Autodesk Fusion 360 part; units mm, degrees
(part 2 of 3)
sketch "Sketch1" plane through (0, 0, 0) normal (0, 0, 1) x (1, 0, 0)
  line L0 (40, 31) -> (-40, 31)
  line L1 (-40, -31) -> (40, -31)
  line L2 (50, 31) -> (-50, -31) construction
  line L3 (-50, 31) -> (50, -31) construction
  line L4 (151, 31) -> (151, 141)
  line L5 (141, 151) -> (60, 151)
  line L6 (50, 141) -> (50, 41)
  line L7 (151, -31) -> (151, -141)
  line L8 (141, -151) -> (60, -151)
  line L9 (50, -141) -> (50, -41)
  line L10 (151, -31) -> (151, 31)
  line L11 (0, 0) -> (0, 31) construction
  line L12 (-141, 151) -> (-60, 151)
  line L13 (-50, 141) -> (-50, 41)
  line L14 (-151, 31) -> (-151, 141)
  line L15 (-151, -31) -> (-151, 31)
  line L16 (-141, -151) -> (-60, -151)
  line L17 (-50, -141) -> (-50, -41)
  line L18 (-151, -31) -> (-151, -141)
  circle A0 centre (0, 0) radius 5
  arc A1 (-141, 151) -> (-151, 141) centre (-141, 141) ccw
  arc A2 (-50, 141) -> (-60, 151) centre (-60, 141) ccw
  arc A3 (60, 151) -> (50, 141) centre (60, 141) ccw
  arc A4 (151, 141) -> (141, 151) centre (141, 141) ccw
  arc A5 (-151, -141) -> (-141, -151) centre (-141, -141) ccw
  arc A6 (-60, -151) -> (-50, -141) centre (-60, -141) ccw
  arc A7 (50, -141) -> (60, -151) centre (60, -141) ccw
  arc A8 (141, -151) -> (151, -141) centre (141, -141) ccw
  arc A9 (-40, -31) -> (-50, -41) centre (-40, -41) ccw
  arc A10 (50, -41) -> (40, -31) centre (40, -41) ccw
  arc A11 (40, 31) -> (50, 41) centre (40, 41) ccw
  arc A12 (-50, 41) -> (-40, 31) centre (-40, 41) ccw
  line L19 (100.5, -151) -> (100.5, -121) construction
  line L20 (119.25, -121) -> (81.75, -121) construction
  circle A13 centre (119.25, -121) radius 1.5
  circle A14 centre (81.75, -121) radius 1.5
  line L21 (151, 0) -> (100, 0) construction
  circle A15 centre (81.75, 121) radius 1.5
  circle A16 centre (119.25, 121) radius 1.5
  line L22 (0, -150) -> (0, -125) construction
  circle A17 centre (-81.75, -121) radius 1.5
  circle A18 centre (-119.25, -121) radius 1.5
  circle A19 centre (-81.75, 121) radius 1.5
  circle A20 centre (-119.25, 121) radius 1.5
  point P0 (50, 151)
  point P1 (50, -151)
  dimension "d1" = 100
  dimension "d2" = 62
  dimension "d3" = 101
  dimension "d4" = 120
  dimension "d5" = 101
  dimension "d6" = 120
  dimension "d9" = 10
  dimension "d10" = 10
  dimension "d11" = 30
  dimension "d12" = 18.75
  dimension "d13" = 37.5
  dimension "d14" = 3
  dimension "d15" = 3
  dimension "d21" = 51
  dimension "d22" = 25
  dimension "d23" = 125
  constraint horizontal L0
  constraint parallel L0 L1
  constraint coincident L2 L11.start
  constraint coincident L3 L11.start
  constraint coincident L11.start A0.centre
  constraint vertical L4
  constraint horizontal L5
  constraint vertical L6
  constraint vertical L7
  constraint horizontal L8
  constraint vertical L9
  constraint symmetric L4.start L11 L14.start
  constraint symmetric L7.start L11 L15.start
  constraint tangent L12 A1
  constraint tangent L14 A1
  constraint tangent L12 A2
  constraint tangent L13 A2
  constraint equal A1 A2
  constraint coincident P0 L5
  constraint coincident P0 L6
  constraint tangent L5 A3
  constraint tangent L6 A3
  constraint equal A1 A3
  constraint tangent L4 A4
  constraint tangent L5 A4
  constraint equal A1 A4
  constraint tangent L16 A5
  constraint tangent L18 A5
  constraint equal A1 A5
  constraint tangent L16 A6
  constraint tangent L17 A6
  constraint equal A1 A6
  constraint coincident P1 L8
  constraint coincident P1 L9
  constraint tangent L8 A7
  constraint tangent L9 A7
  constraint equal A1 A7
  constraint tangent L7 A8
  constraint tangent L8 A8
  constraint equal A1 A8
  constraint coincident L2.end L1
  constraint tangent L1 A9
  constraint tangent L17 A9
  constraint equal A1 A9
  constraint coincident L3.end L1
  constraint coincident L3.end L9
  constraint tangent L1 A10
  constraint tangent L9 A10
  constraint equal A1 A10
  constraint coincident L0 L11.end
  constraint coincident L2.start L6
  constraint coincident L2.start L0
  constraint tangent L6 A11
  constraint tangent L0 A11
  constraint equal A1 A11
  constraint coincident L3.start L0
  constraint tangent L13 A12
  constraint tangent L0 A12
  constraint equal A1 A12
  constraint midpoint L8 L19.start
  constraint perpendicular L8 L19
  constraint coincident L20.start A13.centre
  constraint coincident L20.end A14.centre
  constraint midpoint L10 L21.start
  constraint perpendicular L10 L21
  constraint symmetric A13 L21 A16
  constraint symmetric A14 L21 A15
  constraint vertical L22
  constraint symmetric A13 L22 A18
  constraint symmetric A14 L22 A17
  constraint symmetric A15 L22 A19
  constraint symmetric A16 L22 A20
  constraint parallel L14 L18
  constraint parallel L4 L17
  constraint parallel L1 L12
  constraint parallel L7 L14
  constraint parallel L4 L10
  constraint parallel L4 L13
  constraint parallel L4 L15
  constraint parallel L5 L16
  constraint collinear L5 L12
  constraint collinear L6 L9
  constraint collinear L8 L16
  constraint collinear L11 L22
  constraint collinear L13 L17
  constraint horizontal L20
  constraint vertical L2.end L17.start
  constraint vertical L3.start L17.start
  constraint horizontal L2.start L4.start
  constraint horizontal L19.end A18.centre
  constraint horizontal L11.start L21.end
  measures "d1" distance of L2.end L3.end
  measures "d2" distance of L3.start L2.end
  measures "d3" distance of L2.start L4.start
  measures "d4" distance of L2.start P0
  measures "d5" distance of L3.end L7.start
  measures "d6" distance of L3.end P1
  measures "d9" diameter of A0
  measures "d10" radius of A1
  measures "d11" distance of L19.start L19.end
  measures "d12" distance of L19.end L20.start
  measures "d13" distance of L20.start L20.end
  measures "d14" diameter of A13
  measures "d15" diameter of A14
  measures "d21" distance of L4 L21.end
  measures "d22" vertical distance of L22.start L22.end
  measures "d23" vertical distance of L11.start L22.end
extrude "Extrude1" add sketch "Sketch1" along normal blind 30.6
chamfer "Chamfer1" distance 5.2024 angle 41 1 edges at (-4.6616, 1.8081, 0) measured on face at (4.9938, -0.2492, 20.4)
extrude "Extrude2" cut 1 faces at (-96.5316, 12.7276, 30.6) along direction (0, 0, -1) blind 25.4
equation "d7 = 5.2 mm + 1 in"
equation "d12 = ( 37.5 / 2 ) * 1 mm"

design "FA6 - 12 Gauge 4” Staple Stake"
Autodesk Fusion 360 part; units mm, degrees
sketch "Sketch1" plane through (0, 0, 0) normal (0, 1, 0) x (1, 0, 0)
  line L0 (0, 0) -> (0, -101.6) construction
  line L1 (0, -101.6) -> (16.1278, -101.6)
  line L2 (18.6263, -99.1872) -> (22.09, 0)
  line L3 (18.542, -101.6) -> (48.3661, -101.6) construction
  line L4 (0, 0) -> (22.09, 0) construction
  arc A0 (16.1278, -101.6) -> (18.6263, -99.1872) centre (16.1278, -99.1) ccw
  line L5 (0, -101.6) -> (-16.1278, -101.6)
  arc A1 (-18.6263, -99.1872) -> (-16.1278, -101.6) centre (-16.1278, -99.1) ccw
  line L6 (-18.6263, -99.1872) -> (-22.09, 0)
  line L7 (0, -101.6) -> (-18.75, -101.6) construction
  line L8 (-18.75, -101.6) -> (-18.75, -100.3) construction
  dimension "d1" = 101.6
  dimension "d2" = 18.542
  dimension "d3" = 88
  dimension "d4" = 2.5
  dimension "d13" = 18.75
  dimension "d14" = 1.3
  constraint coincident L0.start L4.start
  constraint vertical L0
  constraint perpendicular L0 L1
  constraint horizontal L3
  constraint perpendicular L0 L4
  constraint coincident L3.start L1
  constraint coincident L3.start L2
  constraint tangent L1 A0
  constraint tangent L2 A0
  constraint symmetric L1.start L0 L5.start
  constraint symmetric L0 L2.end L6.end
  constraint symmetric L0 L1.end L5.end
  constraint symmetric L0 L2.start A1.start
  constraint symmetric L0 A0 A1
  constraint perpendicular L0 L7
  constraint perpendicular L7 L8
  measures "d1" distance of L0.start L0.end
  measures "d2" distance of L0.end L3.start
  measures "d3" angle of L2 L3
  measures "d4" radius of A0
  measures "d13" distance of L0.end L7.end
  measures "d14" distance of L7.end L8.end
sketch "Sketch3" plane through (0, 0, 0) normal (1, 0, 0) x (0, 1, 0)
  line L0 (0, 0) -> (0, 101.6) construction
  circle A0 centre (0, 101.6) radius 1.3
  dimension "d5" = 101.6
  dimension "d6" = 2.6
  constraint coincident L0.start origin
  constraint vertical L0
  constraint coincident L0.end A0.centre
  measures "d5" distance of L0.start L0.end
  measures "d6" diameter of A0
sweep "Sweep1" add profiles "Sketch3" path "Sketch1" along L6 A1 L5 L1 A0 L2 section 1
ref_plane "WorkPlane1" through (0, 0, 100.3) normal (0, 0, 1) x (1, 0, 0)
sketch "Sketch4" plane through (0, 0, 100.3) normal (0, 0, 1) x (1, 0, 0)
  line L0 (0, 0) -> (-18.75, 0) construction
  circle A0 centre (-18.75, 0) radius 5 construction
  dimension "d16" = 18.75
  dimension "d17" = 10
  constraint coincident L0.start origin
  constraint horizontal L0
  constraint coincident L0.end A0.centre
  measures "d16" distance of L0.start L0.end
  measures "d17" diameter of A0
chamfer "Chamfer1" distance 1.3 distance2 4 2 edges at (-22.5598, -1.212, 0.0164) (21.6201, -1.212, -0.0164) measured on face at (-22.2737, 0.4465, 0.0064) measured on face at (22.1502, -0.4097, 0.0021)
equation "d2 = ( 37.084 / 2 ) * 1 mm"
equation "d13 = ( 37.5 / 2 ) * 1 mm"

design "LB2 - Buffer Disk"
Autodesk Fusion 360 part; units mm, degrees
sketch "Sketch1" plane through (0, 0, 0) normal (0, 0, 1) x (1, 0, 0)
  circle A0 centre (0, 0) radius 31
  circle A1 centre (0, 0) radius 5
  dimension "d1" = 62
  dimension "d2" = 10
  constraint coincident A0.centre A1.centre
  constraint concentric A0 A1
  measures "d1" diameter of A0
  measures "d2" diameter of A1
extrude "Extrude1" add sketch "Sketch1" along normal blind 5.2

design "PE4 - PCB Case Lid"
Autodesk Fusion 360 part; units mm, degrees
sketch "Sketch1" plane through (0, 0, 0) normal (0, 0, 1) x (1, 0, 0)
  line L0 (6.2013, 11.75) -> (-6.2012, 11.75)
  line L1 (10.25, 10.25) -> (-10.25, -10.25) construction
  arc A0 (-6.2012, 11.75) -> (-11.75, 6.2013) centre (-6.2013, 6.2013) ccw
  line L2 (-11.75, 6.2013) -> (-11.75, -6.2013)
  arc A1 (-11.75, -6.2012) -> (-6.2012, -11.75) centre (-6.2013, -6.2013) ccw
  line L3 (-6.2012, -11.75) -> (6.2013, -11.75)
  arc A2 (11.75, 6.2012) -> (6.2013, 11.75) centre (6.2012, 6.2012) ccw
  arc A3 (6.2013, -11.75) -> (11.75, -6.2012) centre (6.2013, -6.2013) ccw
  line L4 (-10.25, 10.25) -> (10.25, -10.25) construction
  line L5 (11.75, -6.2012) -> (11.75, 6.2012)
  circle A4 centre (6.2012, 6.2012) radius 1.7
  circle A5 centre (-6.2013, -6.2013) radius 1.7
  line L6 (-6.2013, -6.2013) -> (-6.2013, -4) construction
  line L7 (-6.2013, -6.2013) -> (-4, -6.2013) construction
  line L8 (-4, -6.2013) -> (-4, -10.15)
  line L9 (-6.2013, -4) -> (-10.15, -4)
  line L10 (-4, -6.2013) -> (-4, -5)
  line L11 (-6.2013, -4) -> (-5, -4)
  arc A6 (-4, -5) -> (-5, -4) centre (-5, -5) ccw
  line L12 (6.2013, 4) -> (10.15, 4)
  line L13 (6.2013, 4) -> (5, 4)
  arc A7 (4, 5) -> (5, 4) centre (5, 5) ccw
  line L14 (4, 6.2013) -> (4, 5)
  line L15 (4, 6.2013) -> (4, 10.15)
  line L16 (10.15, -6.2012) -> (10.15, 6.2012)
  arc A8 (10.15, 6.2012) -> (6.2013, 10.15) centre (6.2012, 6.2012) ccw
  line L17 (6.2012, 10.15) -> (-6.2012, 10.15)
  arc A9 (-6.2012, 10.15) -> (-10.15, 6.2013) centre (-6.2013, 6.2013) ccw
  line L18 (-10.15, 6.2013) -> (-10.15, -6.2012)
  arc A10 (-10.15, -6.2012) -> (-6.2012, -10.15) centre (-6.2013, -6.2013) ccw
  line L19 (-6.2012, -10.15) -> (6.2013, -10.15)
  arc A11 (6.2013, -10.15) -> (10.15, -6.2013) centre (6.2013, -6.2013) ccw
  arc A12 (9.15, 6.2012) -> (6.2012, 9.15) centre (6.2012, 6.2012) ccw
  line L20 (6.2012, 9.15) -> (-6.2012, 9.15)
  arc A13 (-6.2012, 9.15) -> (-9.15, 6.2013) centre (-6.2013, 6.2013) ccw
  line L21 (-9.15, 6.2013) -> (-9.15, -6.2012)
  arc A14 (-9.15, -6.2012) -> (-6.2013, -9.15) centre (-6.2013, -6.2013) ccw
  line L22 (-6.2013, -9.15) -> (6.2013, -9.15)
  arc A15 (6.2013, -9.15) -> (9.15, -6.2013) centre (6.2013, -6.2013) ccw
  line L23 (9.15, -6.2013) -> (9.15, 6.2012)
  dimension "d2" = 20.5
  dimension "d3" = 20.5
  dimension "d8" = 3.4
  dimension "d9" = 3.4
  dimension "d13" = 1
  dimension "d26" = -1.6
  dimension "d27" = -2.6
  dimension "d89" = 5
  dimension "d90" = 9
  dimension "d91" = 9
  dimension "d92" = 6.75
  dimension "d93" = 1.2012
  dimension "d94" = 1
  dimension "d95" = 14.15
  dimension "d96" = 6.75
  dimension "d97" = 1.2012
  dimension "d98" = 14.15
  dimension "d99" = 2.2012
  dimension "d100" = 2.2012
  dimension "d101" = 2.2012
  dimension "d102" = 2.2012
  dimension "d103" = 135
  dimension "d104" = 5
  constraint coincident origin L1
  constraint coincident origin L4
  constraint vertical L6
  constraint perpendicular L6 L7
  constraint perpendicular L6 L9
  constraint perpendicular L7 L10
  constraint perpendicular L10 L11
  constraint tangent L10 A6
  constraint tangent L11 A6
  constraint vertical L15
  constraint horizontal L12
  constraint coincident L8.end L19
  constraint perpendicular L8 L19
  constraint coincident L9.end L18
  constraint perpendicular L9 L18
  constraint coincident L15.end L17
  constraint perpendicular L15 L17
  constraint coincident L12.end L16
  constraint perpendicular L12 L16
  constraint tangent A7 L14
  constraint tangent L13 A7
  constraint equal A6 A7
  constraint tangent A0 L2
  constraint tangent L0 A0
  constraint equal A0 A1
  constraint equal A0 A2
  constraint equal A0 A3
  constraint equal L10 L13
  constraint equal L10 L14
  constraint parallel L14 L15
  constraint parallel L12 L13
  constraint vertical L12.start L22.end
  constraint horizontal L14.start A12.start
  constraint midpoint origin L1
  constraint tangent L2 A1
  constraint equal L0 L2
  constraint equal L0 L18
  constraint equal L0 L21
  constraint equal L6 L7
  constraint equal L0 L23
  constraint equal L0 L16
  constraint equal L0 L5
  constraint tangent A1 L3
  constraint equal L0 L3
  constraint equal L0 L19
  constraint equal L0 L22
  constraint concentric A2 A4
  constraint concentric A1 A5
  constraint vertical L1.end L4.start
  constraint vertical L1.start L4.end
  constraint coincident A1.centre A5.centre
  measures "d2" distance of L1.start L4.start
  measures "d3" distance of L1.start L4.end
  measures "d8" diameter of A4
  measures "d9" diameter of A5
  measures "d13" radius of A6
  measures "d89" horizontal distance of origin A6.centre
  measures "d90" distance of A6.centre L13
  measures "d91" distance of A6.centre L14
  measures "d92" distance of L2 A6.centre
  measures "d93" distance of L6 A6.centre
  measures "d94" distance of L8 A6.centre
  measures "d95" distance of A6.centre L23
  measures "d96" distance of L3 A6.centre
  measures "d97" distance of L7 A6.centre
  measures "d98" distance of A6.centre L20
  measures "d99" distance of A0.centre L10
  measures "d100" distance of A3.centre L11
  measures "d101" distance of A2.centre L14
  measures "d102" distance of A2.centre L12
  measures "d103" angle of L1 L9
  measures "d104" vertical distance of origin A6.centre
sketch "Sketch2" plane through (0, 0, 0) normal (0, 0, 1) x (1, 0, 0)
  line L0 (-6.2013, -27.25) -> (6.2012, -27.25)
  arc A0 (6.2012, -27.25) -> (12.25, -21.2012) centre (6.2013, -21.2012) ccw
  line L1 (12.25, -21.2012) -> (12.25, 21.2013)
  arc A1 (12.25, 21.2013) -> (6.2013, 27.25) centre (6.2012, 21.2013) ccw
  line L2 (6.2013, 27.25) -> (-6.2012, 27.25)
  arc A2 (-6.2012, 27.25) -> (-12.25, 21.2013) centre (-6.2013, 21.2013) ccw
  line L3 (-12.25, 21.2013) -> (-12.25, -21.2012)
  arc A3 (-12.25, -21.2012) -> (-6.2013, -27.25) centre (-6.2013, -21.2012) ccw
  line L4 (-10.15, 21.2013) -> (-10.15, -21.2012)
  arc A4 (-10.15, -21.2012) -> (-6.2013, -25.15) centre (-6.2013, -21.2012) ccw
  line L5 (-6.2013, -25.15) -> (6.2013, -25.15)
  arc A5 (6.2013, -25.15) -> (10.15, -21.2012) centre (6.2013, -21.2012) ccw
  line L6 (10.15, -21.2012) -> (10.15, 17.8428)
  line L7 (2.8428, 25.15) -> (-6.2013, 25.15)
  arc A6 (-6.2013, 25.15) -> (-10.15, 21.2013) centre (-6.2013, 21.2013) ccw
  circle A7 centre (6.9428, 21.9428) radius 1.6
  circle A8 centre (-6.9428, -21.9428) radius 1.6
  line L8 (-6.2013, -25.15) -> (6.2012, -25.15)
  arc A9 (6.2012, -25.15) -> (10.15, -21.2012) centre (6.2013, -21.2012) ccw
  line L9 (10.15, -21.2012) -> (10.15, 21.2013)
  arc A10 (10.15, 21.2013) -> (6.2013, 25.15) centre (6.2012, 21.2013) ccw
  line L10 (6.2013, 25.15) -> (-6.2012, 25.15)
  arc A11 (-6.2012, 25.15) -> (-10.15, 21.2013) centre (-6.2013, 21.2013) ccw
  line L11 (-10.15, 21.2013) -> (-10.15, -21.2012)
  arc A12 (-10.15, -21.2012) -> (-6.2013, -25.15) centre (-6.2013, -21.2012) ccw
  line L12 (2.8428, 23.65) -> (-6.2013, 23.65)
  arc A13 (-6.2013, 23.65) -> (-8.65, 21.2013) centre (-6.2013, 21.2013) ccw
  line L13 (-8.65, 21.2013) -> (-8.65, -17.8428)
  line L14 (2.8428, 25.15) -> (2.8428, 23.65)
  line L15 (-8.65, -17.8428) -> (-10.15, -17.8428)
  line L16 (-2.8428, -23.65) -> (6.2013, -23.65)
  arc A14 (6.2013, -23.65) -> (8.65, -21.2012) centre (6.2013, -21.2012) ccw
  line L17 (8.65, -21.2012) -> (8.65, 17.8428)
  line L18 (-2.8428, -25.15) -> (-2.8428, -23.65)
  line L19 (10.15, 17.8428) -> (8.65, 17.8428)
  dimension "d62" = 3.2
  dimension "d63" = 3.2
  dimension "d71" = -2.1
  dimension "d105" = 8.65
  dimension "d106" = 17.8428
  dimension "d107" = 1.7072
  dimension "d108" = 15.5928
  dimension "d109" = 4.1
  dimension "d110" = 39.7857
  dimension "d111" = 6.0488
  dimension "d112" = 1.5
  dimension "d113" = 39.0441
  dimension "d114" = 2.4487
  dimension "d115" = 2.4488
  dimension "d116" = 5.8072
  dimension "d117" = 11.4928
  dimension "d118" = 14.8513
  dimension "d119" = 17.3
  dimension "d120" = 18.8
  dimension "d121" = 9.4072
  dimension "d122" = 5.8072
  dimension "d123" = 35.6857
  dimension "d124" = 7.3072
  dimension "d125" = 22.4
  dimension "d126" = 1.5
  constraint coincident L5 L18.start
  constraint perpendicular L7 L14
  constraint perpendicular L11 L15
  constraint coincident L4 L15.end
  constraint perpendicular L16 L18
  constraint perpendicular L17 L19
  constraint tangent A14 L17
  constraint tangent A13 L13
  constraint tangent L7 A11
  constraint tangent L3 A3
  constraint tangent L0 A3
  constraint tangent A2 L3
  constraint tangent L2 A2
  constraint tangent A1 L2
  constraint tangent L1 A1
  constraint tangent L0 A0
  constraint tangent A0 L1
  constraint concentric A6 A11
  constraint concentric A11 A13
  constraint concentric A3 A4
  constraint concentric A0 A5
  constraint coincident L4.start A11
  constraint perpendicular L13 L15
  constraint perpendicular L4 L15
  constraint equal A0 A3
  constraint equal A0 A2
  constraint equal A0 A1
  constraint equal L6 L13
  constraint equal L14 L15
  constraint midpoint A6 A11
  constraint midpoint L4 L11
  constraint parallel L0 L12
  constraint equal L7 L16
  measures "d62" diameter of A7
  measures "d63" diameter of A8
  measures "d105" distance of origin L13
  measures "d106" distance of origin L15
  measures "d107" distance of A8.centre L13
  measures "d108" distance of A7.centre L13
  measures "d109" distance of A8.centre L15
  measures "d110" distance of A7.centre L15
  measures "d111" radius of A2
  measures "d112" distance of L4.start L13
  measures "d113" distance of L1.end L15
  measures "d114" distance of L0.start L13
  measures "d115" distance of L2.end L13
  measures "d116" distance of L13 L18
  measures "d117" distance of L13 L14
  measures "d118" distance of A1.end L13
  measures "d119" distance of L13 L17
  measures "d120" distance of L9 L13
  measures "d121" distance of L0 L15
  measures "d122" distance of L15 L16
  measures "d123" distance of L15 L19
  measures "d124" distance of L18.start L15
  measures "d125" distance of L3 L6
  measures "d126" distance of A5 A14
extrude "Extrude5" add sketch "Sketch2" along normal blind 5 contours L0 A0 L1 A1 L2 A2 L3 A3 | L4 L7 A6 L10 A11 L11 L12 A13 L13 L14 L15 | L4 A4 L5 L8 L9 A10 L10 L11 A12 L12 A13 L13 L14 L15 L16 A14 L17 L18 L19 | L5 A5 L6 L8 A9 L9 L16 A14 L17 L18 L19 | A7 | A8
extrude "Extrude6" add sketch "Sketch2" against normal blind 2 contours L4 L7 A6 L10 A11 L11 L12 A13 L13 L14 L15 | L5 A5 L6 L8 A9 L9 L16 A14 L17 L18 L19
sketch "Sketch3" plane through (0, 0, 0) normal (0, 1, 0) x (1, 0, 0)
  line L0 (1.7, 3) -> (1.7, 0) construction
  line L1 (-0.45, 0) -> (-0.45, 2.15)
  line L2 (3.85, -0.0044) -> (3.85, 2.1456)
  line L3 (-0.45, 2.15) -> (3.85, 2.1456)
  arc A0 (1.7991, 2.1477) -> (1.6052, 2.1479) centre (1.7, 0) ccw
  arc A1 (-0.45, 0) -> (3.85, 0.0044) centre (1.7, 0) ccw
  line L4 (5.2, -5) -> (-1.8, -5)
  line L5 (-1.8, -5) -> (-1.8, 0)
  line L6 (5.2, 0) -> (5.2, -5)
  line L7 (5.2, -5) -> (0.1955, 2.1493) construction
  line L8 (-1.8, -5) -> (3.2024, 2.1463) construction
  line L9 (5.2, 0) -> (3.85, 0)
  line L10 (-0.45, 0) -> (-1.8, 0)
  point P0 (1.7, 0)
  dimension "d45" = 2.15
  dimension "d46" = 2.15
  dimension "d127" = 2.15
  dimension "d128" = 3.5
  dimension "d129" = 3.5
  dimension "d130" = 2.15
  dimension "d131" = 1.5045
  dimension "d132" = 1.5024
  dimension "d133" = 0.45
  dimension "d134" = 8
  constraint vertical L0
  constraint coincident L1.start A0
  constraint vertical L1
  constraint coincident L2.start A0
  constraint vertical L2
  constraint coincident L2 A1.end
  constraint coincident L3 A0.start
  constraint coincident L3 A0.end
  constraint concentric A0 A1
  constraint horizontal L4
  constraint perpendicular L4 L5
  constraint parallel L5 L6
  constraint coincident L7 P0
  constraint coincident L8 P0
  constraint coincident P0 L0.end
  constraint horizontal L9
  constraint coincident L3 L8.end
  constraint coincident L3 L7.end
  constraint coincident L2 L9.end
  constraint collinear L9 L10
  constraint horizontal origin L1.start
  constraint tangent L1 A1
  measures "d45" distance of L1.start L1.end
  measures "d46" distance of L2.start L2.end
  measures "d127" radius of A1
  measures "d128" distance of L0 L5
  measures "d129" distance of L0 L6
  measures "d130" distance of L0 L2
  measures "d131" distance of L0 L7.end
  measures "d132" distance of L0 L8.end
  measures "d133" distance of origin L1
  measures "d134" distance of L0.start L4
extrude "Extrude7" cut sketch "Sketch2" along normal blind 3 contours L4 A4 L5 L8 L9 A10 L10 L11 A12 L12 A13 L13 L14 L15 L16 A14 L17 L18 L19 | A7 | A8
extrude "Extrude8" cut sketch "Sketch3" against normal blind 31 contours L1 L2 L3 A0 A1
extrude "Extrude9" add sketch "Sketch3" against normal blind 8 from surface at -27.25 contours L2 A1 L4 L5 L6 L9 L10
sketch "Sketch4" plane through (0, 0, 0) normal (0, 1, 0) x (1, 0, 0)
  line L0 (6.2012, 4) -> (6.2, 4)
  line L1 (-6.2013, 0) -> (0.8, 0)
  line L2 (-4.85, 0) -> (-4.85, 2.15)
  line L3 (-4.85, 2.15) -> (-0.55, 2.1456)
  line L4 (-0.55, -0.0044) -> (-0.55, 2.1456)
  line L5 (-4.85, 0) -> (-2.7, 0) construction
  arc A0 (-4.85, 0) -> (-0.55, 0.0044) centre (-2.7, 0) ccw
  arc A1 (-2.6009, 2.1477) -> (-2.7948, 2.1479) centre (-2.7, 0) ccw
  line L6 (-6.2, -5) -> (0.8, -5)
  line L7 (0.8, -5) -> (0.8, 0)
  line L8 (-6.2, 0) -> (-6.2, -5)
  line L9 (-6.2, -5) -> (-1.1976, 2.1463) construction
  line L10 (0.8, -5) -> (-4.2045, 2.1493) construction
  line L11 (-4.85, 0) -> (-6.2013, 0)
  line L12 (-0.55, -0.0044) -> (0.8, 0)
  point P0 (-2.7, 0)
  dimension "d53" = 2.15
  dimension "d54" = 2.15
  dimension "d55" = 2.15
  dimension "d135" = 0.55
  dimension "d136" = 6.75
  dimension "d137" = 2.15
  dimension "d138" = 0.0044
  dimension "d139" = 1.35
  dimension "d140" = 4.9956
  dimension "d141" = 5.65
  dimension "d142" = 6.7513
  dimension "d143" = 4
  dimension "d144" = 5.6512
  constraint horizontal L1
  constraint horizontal L0
  constraint vertical L2
  constraint vertical L4
  constraint perpendicular L2 L5
  constraint coincident L3 A1.end
  constraint coincident L4 A0.end
  constraint coincident L3 A1.start
  constraint concentric A0 A1
  constraint horizontal L6
  constraint perpendicular L6 L7
  constraint parallel L7 L8
  constraint coincident L9 P0
  constraint coincident L10 P0
  constraint coincident P0 L5.end
  constraint perpendicular L8 L11
  constraint coincident L3 L9.end
  constraint coincident L3 L10.end
  constraint coincident L1 L8.start
  constraint tangent L2 A0
  constraint coincident L4.start A0
  constraint equal A0 A1
  constraint coincident origin L1
  measures "d53" distance of L2.start L2.end
  measures "d54" distance of L3.end L4.start
  measures "d55" distance of L2.start P0
  measures "d135" distance of origin L4
  measures "d136" distance of L0.end L4
  measures "d137" radius of A0
  measures "d138" distance of L4.start L5
  measures "d139" distance of L4 L7
  measures "d140" distance of L4.start L6
  measures "d141" distance of L4 L8
  measures "d142" distance of L0.start L4
  measures "d143" distance of L0 L11
  measures "d144" distance of L1.start L4
extrude "Extrude10" add sketch "Sketch4" along normal blind 8 from surface at 27.25 contours L1 A0 L6 L7 L8 L11 L12
extrude "Extrude11" cut sketch "Sketch4" along normal blind 61 contours L1 L2 L3 L4 A0 A1 | L1 L4 A0
extrude "Extrude12" cut sketch "Sketch2" along normal blind 20 contours A7 | A8
extrude "Extrude13" add 1 faces at (-4.3101, 7.137, 5) along direction (0, 0, 1) blind 2
sketch "Sketch5" plane through (0, 0, 3) normal (0, 0, -1) x (1, 0, 0)
  circle A0 centre (6.9428, -21.9428) radius 1.6
  circle A1 centre (-6.9428, 21.9428) radius 1.6
  arc A2 (-6.2013, 25.15) -> (-10.15, 21.2012) centre (-6.2013, 21.2012) ccw
  line L0 (-10.15, 21.2012) -> (-10.15, 17.8428)
  line L1 (2.8428, -25.15) -> (6.2013, -25.15)
  arc A3 (6.2013, -25.15) -> (10.15, -21.2013) centre (6.2012, -21.2013) ccw
  line L2 (10.15, -21.2013) -> (10.15, -17.8428)
  line L3 (9.15, -17.8428) -> (-9.15, -17.8428)
  line L4 (-9.15, -17.8428) -> (-9.15, 17.8428)
  line L5 (-9.15, 17.8428) -> (9.15, 17.8428)
  line L6 (9.15, 17.8428) -> (9.15, -17.8428)
  line L7 (-10.15, 17.8428) -> (-8.65, 17.8428)
  line L8 (-8.65, 17.8428) -> (-8.65, -21.2013)
  arc A4 (-8.65, -21.2013) -> (-6.2013, -23.65) centre (-6.2013, -21.2013) ccw
  line L9 (-6.2013, -23.65) -> (2.8428, -23.65)
  line L10 (2.8428, -23.65) -> (2.8428, -25.15)
  line L11 (10.15, -17.8428) -> (8.65, -17.8428)
  line L12 (8.65, -17.8428) -> (8.65, 21.2012)
  arc A5 (8.65, 21.2012) -> (6.2013, 23.65) centre (6.2013, 21.2012) ccw
  line L13 (6.2013, 23.65) -> (-2.8428, 23.65)
  line L14 (-2.8428, 23.65) -> (-2.8428, 25.15)
  line L15 (-2.8428, 25.15) -> (-6.2013, 25.15)
  dimension "d145" = 1
  dimension "d146" = 18.3
  constraint horizontal L3
  constraint vertical L4
  constraint horizontal L5
  constraint vertical L6
  constraint coincident L3.start L11
  constraint coincident L4.end L7
  measures "d145" distance of L0.end L4
  measures "d146" distance of L4 L6
extrude "Extrude14" cut sketch "Sketch5" against normal blind 2 contours L3 L4 L5 L7 L8 | L3 L5 L8 L12 | L3 L5 L6 L11 L12
sketch "Sketch6" plane through (0, 0, 5) normal (0, 0, -1) x (1, 0, 0)
  line L0 (9.15, 17.8428) -> (-9.15, 17.8428)
  line L1 (-9.15, 17.8428) -> (-9.15, -17.8428)
  line L2 (-9.15, -17.8428) -> (9.15, -17.8428)
  line L3 (9.15, -17.8428) -> (9.15, 17.8428)
  line L4 (6.2012, -6.2012) -> (6.2012, -3.7012) construction
  line L5 (6.2012, -3.7012) -> (9.15, -3.7012)
  line L6 (9.15, -8.7012) -> (6.2012, -8.7012)
  arc A0 (6.2012, -3.7012) -> (6.2012, -8.7012) centre (6.2012, -6.2012) ccw
  line L7 (-6.2013, 3.7013) -> (-9.15, 3.7013)
  line L8 (-9.15, 8.7013) -> (-6.2013, 8.7013)
  arc A1 (-6.2013, 3.7013) -> (-6.2013, 8.7013) centre (-6.2013, 6.2013) ccw
  line L9 (-9.15, 3.7013) -> (-10.15, 3.7013)
  line L10 (-10.15, 3.7013) -> (-10.15, 8.7013)
  line L11 (-10.15, 8.7013) -> (-9.15, 8.7013)
  line L12 (9.15, -8.7012) -> (10.15, -8.7012)
  line L13 (10.15, -8.7012) -> (10.15, -3.7012)
  line L14 (10.15, -3.7012) -> (9.15, -3.7012)
  dimension "d75" = 5
  dimension "d76" = 5
  dimension "d79" = 1
  dimension "d80" = 5
  dimension "d81" = 1
  dimension "d82" = 5
  dimension "d147" = 15.3512
  dimension "d148" = 21.5441
  dimension "d149" = 14.1416
  constraint coincident L4.start A0.centre
  constraint parallel L5 L6
  constraint parallel L7 L8
  constraint horizontal L9
  constraint vertical L10
  constraint horizontal L11
  constraint horizontal L12
  constraint vertical L13
  constraint horizontal L14
  constraint tangent L7 A1
  constraint tangent L8 A1
  constraint tangent L6 A0
  constraint tangent L5 A0
  constraint coincident L1 L7.end
  constraint coincident L1 L8.start
  constraint coincident L3 L5.end
  constraint coincident L3 L6.start
  constraint equal L5 L7
  measures "d75" diameter of A1
  measures "d76" diameter of A0
  measures "d79" distance of L7.end L9.end
  measures "d80" distance of L7.end L8.start
  measures "d81" distance of L6.start L12.end
  measures "d82" distance of L6.start L5.end
  measures "d147" distance of L1 L4
  measures "d148" distance of L2 L7
  measures "d149" distance of L2 L5
extrude "Extrude15" add sketch "Sketch6" along normal blind 12.45 contours L3 L12 L13 L14 | L3 L5 L6 A0 | L1 L7 L8 A1 | L1 L9 L10 L11
extrude "Extrude16" add 1 faces at (-2.0372, -23.65, 0.4401) along direction (0, 1, 0) blind 2
extrude "Extrude17" add 1 faces at (1.7037, 23.65, 0.4415) along direction (0, -1, 0) blind 2
equation "d45 = ( 4.3 / 2 ) * 1 mm"
equation "d46 = ( 4.3 / 2 ) * 1 mm"
equation "d53 = ( 4.3 / 2 ) * 1 mm"
equation "d54 = ( 4.3 / 2 ) * 1 mm"
equation "d55 = ( 4.3 / 2 ) * 1 mm"
equation "d77 = 5.00 mm + 7.45 mm"

design "Top Component (FA1)"
Autodesk Fusion 360 part; units mm, degrees
sketch "Sketch1" plane through (0, 0, 0) normal (0, 0, 1) x (1, 0, 0)
  circle A0 centre (0, 0) radius 110
  circle A1 centre (0, 0) radius 106.5
  arc A2 (10.2564, 113.75) -> (12.5979, 109.2762) centre (20, 116) ccw
  arc A3 (9.7436, 118.25) -> (-10, 116) centre (0, 116) ccw
  arc A4 (-12.5979, 109.2762) -> (-10, 116) centre (-20, 116) ccw
  line L0 (0, 113.75) -> (10.2564, 113.75)
  line L1 (9.7436, 118.25) -> (0, 118.25)
  arc A5 (0, 118.25) -> (0, 113.75) centre (0, 116) ccw
  line L2 (12.5979, 109.2762) -> (12.5979, 107)
  line L3 (12.5979, 107) -> (-12.5979, 107)
  line L4 (-12.5979, 107) -> (-12.5979, 109.2762)
  dimension "d1" = 220
  dimension "d2" = 213
  dimension "d41" = 4.5
  dimension "d54" = 7.75
  dimension "d55" = 12.5979
  dimension "d56" = 107
  dimension "d57" = 11.25
  dimension "d58" = 40
  dimension "d59" = 10.2564
  constraint coincident A0.centre A1.centre
  constraint concentric A0 A1
  constraint parallel L0 L1
  constraint vertical L2
  constraint perpendicular L2 L3
  constraint perpendicular L3 L4
  constraint tangent L0 A5
  constraint tangent L1 A5
  constraint concentric A3 A5
  constraint coincident A0 A2.end
  constraint vertical A0.centre L0.start
  constraint equal A2 A3
  constraint equal A2 A4
  constraint coincident A3.end A4.end
  constraint parallel L0 L3
  constraint equal L2 L4
  measures "d1" diameter of A0
  measures "d2" diameter of A1
  measures "d41" diameter of A5
  measures "d54" distance of A3 A5
  measures "d55" distance of A0.centre L4
  measures "d56" distance of A0.centre L3
  measures "d57" distance of A3.start L3
  measures "d58" horizontal distance of A4.centre A2.centre
  measures "d59" distance of L0.start A2.start
ref_plane "WorkPlane1" through (0, 0, 220) normal (0, 0, 1) x (1, 0, 0)
sketch "Sketch2" plane through (0, 0, 220) normal (0, 0, 1) x (1, 0, 0)
  circle A0 centre (0, 0) radius 105
  circle A1 centre (0, 0) radius 101.5
  dimension "d4" = 210
  dimension "d5" = 203
  constraint coincident A0.centre A1.centre
  measures "d4" diameter of A0
  measures "d5" diameter of A1
sketch "Sketch3" plane through (0, 0, 0) normal (0, 1, 0) x (1, 0, 0)
  line L0 (0, 0) -> (-110, 0) construction
  line L1 (-110, 0) -> (-106.5, 0)
  line L2 (0, -200) -> (-105, -200) construction
  line L3 (-105, -200) -> (-101.5, -200)
  line L4 (-105, -200) -> (-110, 0)
  line L5 (-106.5, 0) -> (-101.5, -200)
  line L6 (0, 0) -> (0, -10) construction
  line L7 (0, -10) -> (0, -200) construction
  dimension "d6" = 110
  dimension "d7" = 3.5
  dimension "d8" = 105
  dimension "d9" = 3.5
  dimension "d42" = 190
  dimension "d60" = 200
  constraint coincident L0.start L6.start
  constraint horizontal L0
  constraint parallel L0 L1
  constraint horizontal L2
  constraint parallel L2 L3
  constraint perpendicular L0 L6
  constraint perpendicular L0 L7
  constraint coincident L2.start L7.end
  measures "d6" distance of L0.start L0.end
  measures "d7" distance of L0.end L1.end
  measures "d8" distance of L2.start L2.end
  measures "d9" distance of L2.end L3.end
  measures "d42" distance of L6.end L2.start
  measures "d60" distance of L0 L2
revolve "Revolve1" add sketch "Sketch3" angle 360 about axis through (0, 0, 1.75) along (0, 0, 1) makes body 1
extrude "Extrude1" add sketch "Sketch1" along normal blind 4 contours A0 L2 L3 L4 | A0 A2 A3 A4 L0 L1 A5 picked at (1.4025, 107.9732) bodies 1
pattern_circular "C-Pattern1" count 4 over 360 about axis through (0, 0, 1.75) along (0, 0, 1) of "Extrude1"
ref_plane "WorkPlane2" through (0, 0, 110) normal (0, 0, 1) x (1, 0, 0)
sketch "Sketch5" plane through (0, 0, 0) normal (0, 1, 0) x (-1, 0, 0)
  line L0 (-30, 114) -> (-103.6332, 140.8003)
  line L1 (-0.0018, 113.6676) -> (57.7728, 113.6676) construction
  line L2 (-103.6332, 140.8003) -> (-106.3694, 133.2828)
  line L3 (-106.3694, 133.2828) -> (-31.4106, 106)
  line L4 (-30, 114) -> (-30, 106)
  line L5 (-30, 106) -> (-31.4106, 106)
  line L6 (0, 0) -> (0, 110) construction
  point P0 (-30, 110)
  dimension "d47" = 30
  dimension "d49" = 160
  dimension "d50" = 8
  dimension "d51" = 8
  dimension "d52" = 110
  dimension "d61" = 0.3324
  dimension "d62" = 34.8003
  dimension "d63" = 57.7746
  constraint horizontal L1
  constraint perpendicular L0 L2
  constraint parallel L0 L3
  constraint perpendicular L4 L5
  constraint coincident L6.start origin
  constraint perpendicular L1 L6
  constraint midpoint L4 P0
  constraint vertical L4.end P0
  measures "d47" distance of L1.start L0.start
  measures "d49" angle of L0 L1
  measures "d50" distance of L0.end L2.end
  measures "d51" distance of L0.start L4.end
  measures "d52" distance of L6.start L6.end
  measures "d61" distance of L0.start L1
  measures "d62" vertical distance of L0.end L3.end
  measures "d63" horizontal distance of L1.start L1.end
sketch "Sketch4" plane through (0, 0, 110) normal (0, 0, 1) x (1, 0, 0)
  circle A0 centre (0, 0) radius 105.125
  circle A1 centre (0, 0) radius 30
  line L0 (2.5, 2.5) -> (-2.5, 2.5)
  line L1 (-2.5, 2.5) -> (-2.5, -2.5)
  line L2 (-2.5, -2.5) -> (2.5, -2.5)
  line L3 (2.5, -2.5) -> (2.5, 2.5)
  line L4 (2.5, 2.5) -> (-2.5, -2.5) construction
  line L5 (-2.5, 2.5) -> (2.5, -2.5) construction
  line L6 (-10, -27.5) -> (-10, -28.2843)
  line L7 (-5, -27.5) -> (-10, -27.5)
  line L8 (-5, -29.5804) -> (-5, -27.5)
  line L9 (-2.5, -27.5) -> (-2.5, -29.8957)
  line L10 (2.5, -27.5) -> (-2.5, -27.5)
  line L11 (2.5, -29.8957) -> (2.5, -27.5)
  line L12 (5, -27.5) -> (5, -29.5804)
  line L13 (10, -27.5) -> (5, -27.5)
  line L14 (10, -28.2843) -> (10, -27.5)
  line L15 (-20, -20) -> (-22.3607, -20)
  line L16 (-20, -22.3607) -> (-20, -20)
  line L17 (-17.5, -20) -> (-17.5, -24.367)
  line L18 (-16.5831, -25) -> (-12.5, -25)
  line L19 (-12.5, -20) -> (-17.5, -20)
  line L20 (-12.5, -25) -> (-12.5, -20)
  line L21 (-10, -20) -> (-10, -25)
  line L22 (-10, -25) -> (-5, -25)
  line L23 (-5, -20) -> (-10, -20)
  line L24 (-5, -25) -> (-5, -20)
  line L25 (-2.5, -20) -> (-2.5, -25)
  line L26 (-2.5, -25) -> (2.5, -25)
  line L27 (2.5, -20) -> (-2.5, -20)
  line L28 (2.5, -25) -> (2.5, -20)
  line L29 (5, -20) -> (5, -25)
  line L30 (5, -25) -> (10, -25)
  line L31 (10, -20) -> (5, -20)
  line L32 (10, -25) -> (10, -20)
  line L33 (12.5, -20) -> (12.5, -25)
  line L34 (12.5, -25) -> (16.5831, -25)
  line L35 (17.5, -20) -> (12.5, -20)
  line L36 (17.5, -24.367) -> (17.5, -20)
  line L37 (20, -20) -> (20, -22.3607)
  line L38 (22.3607, -20) -> (20, -20)
  line L39 (-25, -12.5) -> (-25, -16.5831)
  line L40 (-24.367, -17.5) -> (-20, -17.5)
  line L41 (-20, -12.5) -> (-25, -12.5)
  line L42 (-20, -17.5) -> (-20, -12.5)
  line L43 (-17.5, -12.5) -> (-17.5, -17.5)
  line L44 (-17.5, -17.5) -> (-12.5, -17.5)
  line L45 (-12.5, -12.5) -> (-17.5, -12.5)
  line L46 (-12.5, -17.5) -> (-12.5, -12.5)
  line L47 (-10, -12.5) -> (-10, -17.5)
  line L48 (-10, -17.5) -> (-5, -17.5)
  line L49 (-5, -12.5) -> (-10, -12.5)
  line L50 (-5, -17.5) -> (-5, -12.5)
  line L51 (-2.5, -12.5) -> (-2.5, -17.5)
  line L52 (-2.5, -17.5) -> (2.5, -17.5)
  line L53 (2.5, -12.5) -> (-2.5, -12.5)
  line L54 (2.5, -17.5) -> (2.5, -12.5)
  line L55 (5, -12.5) -> (5, -17.5)
  line L56 (5, -17.5) -> (10, -17.5)
  line L57 (10, -12.5) -> (5, -12.5)
  line L58 (10, -17.5) -> (10, -12.5)
  line L59 (12.5, -12.5) -> (12.5, -17.5)
  line L60 (12.5, -17.5) -> (17.5, -17.5)
  line L61 (17.5, -12.5) -> (12.5, -12.5)
  line L62 (17.5, -17.5) -> (17.5, -12.5)
  line L63 (20, -12.5) -> (20, -17.5)
  line L64 (20, -17.5) -> (24.367, -17.5)
  line L65 (25, -12.5) -> (20, -12.5)
  line L66 (25, -16.5831) -> (25, -12.5)
  line L67 (-28.2843, -10) -> (-27.5, -10)
  line L68 (-27.5, -5) -> (-29.5804, -5)
  line L69 (-27.5, -10) -> (-27.5, -5)
  line L70 (-25, -5) -> (-25, -10)
  line L71 (-25, -10) -> (-20, -10)
  line L72 (-20, -5) -> (-25, -5)
  line L73 (-20, -10) -> (-20, -5)
  line L74 (-17.5, -5) -> (-17.5, -10)
  line L75 (-17.5, -10) -> (-12.5, -10)
  line L76 (-12.5, -5) -> (-17.5, -5)
  line L77 (-12.5, -10) -> (-12.5, -5)
  line L78 (-10, -5) -> (-10, -10)
  line L79 (-10, -10) -> (-5, -10)
  line L80 (-5, -5) -> (-10, -5)
  line L81 (-5, -10) -> (-5, -5)
  line L82 (-2.5, -5) -> (-2.5, -10)
  line L83 (-2.5, -10) -> (2.5, -10)
  line L84 (2.5, -5) -> (-2.5, -5)
  line L85 (2.5, -10) -> (2.5, -5)
  line L86 (5, -5) -> (5, -10)
  line L87 (5, -10) -> (10, -10)
  line L88 (10, -5) -> (5, -5)
  line L89 (10, -10) -> (10, -5)
  line L90 (12.5, -5) -> (12.5, -10)
  line L91 (12.5, -10) -> (17.5, -10)
  line L92 (17.5, -5) -> (12.5, -5)
  line L93 (17.5, -10) -> (17.5, -5)
  line L94 (20, -5) -> (20, -10)
  line L95 (20, -10) -> (25, -10)
  line L96 (25, -5) -> (20, -5)
  line L97 (25, -10) -> (25, -5)
  line L98 (27.5, -5) -> (27.5, -10)
  line L99 (27.5, -10) -> (28.2843, -10)
  line L100 (29.5804, -5) -> (27.5, -5)
  line L101 (-29.8957, -2.5) -> (-27.5, -2.5)
  line L102 (-27.5, 2.5) -> (-29.8957, 2.5)
  line L103 (-27.5, -2.5) -> (-27.5, 2.5)
  line L104 (-25, 2.5) -> (-25, -2.5)
  line L105 (-25, -2.5) -> (-20, -2.5)
  line L106 (-20, 2.5) -> (-25, 2.5)
  line L107 (-20, -2.5) -> (-20, 2.5)
  line L108 (-17.5, 2.5) -> (-17.5, -2.5)
  line L109 (-17.5, -2.5) -> (-12.5, -2.5)
  line L110 (-12.5, 2.5) -> (-17.5, 2.5)
  line L111 (-12.5, -2.5) -> (-12.5, 2.5)
  line L112 (-10, 2.5) -> (-10, -2.5)
  line L113 (-10, -2.5) -> (-5, -2.5)
  line L114 (-5, 2.5) -> (-10, 2.5)
  line L115 (-5, -2.5) -> (-5, 2.5)
  line L116 (5, 2.5) -> (5, -2.5)
  line L117 (5, -2.5) -> (10, -2.5)
  line L118 (10, 2.5) -> (5, 2.5)
  line L119 (10, -2.5) -> (10, 2.5)
  line L120 (12.5, 2.5) -> (12.5, -2.5)
  line L121 (12.5, -2.5) -> (17.5, -2.5)
  line L122 (17.5, 2.5) -> (12.5, 2.5)
  line L123 (17.5, -2.5) -> (17.5, 2.5)
  line L124 (20, 2.5) -> (20, -2.5)
  line L125 (20, -2.5) -> (25, -2.5)
  line L126 (25, 2.5) -> (20, 2.5)
  line L127 (25, -2.5) -> (25, 2.5)
  line L128 (27.5, 2.5) -> (27.5, -2.5)
  line L129 (27.5, -2.5) -> (29.8957, -2.5)
  line L130 (29.8957, 2.5) -> (27.5, 2.5)
  line L131 (-29.5804, 5) -> (-27.5, 5)
  line L132 (-27.5, 10) -> (-28.2843, 10)
  line L133 (-27.5, 5) -> (-27.5, 10)
  line L134 (-25, 10) -> (-25, 5)
  line L135 (-25, 5) -> (-20, 5)
  line L136 (-20, 10) -> (-25, 10)
  line L137 (-20, 5) -> (-20, 10)
  line L138 (-17.5, 10) -> (-17.5, 5)
  line L139 (-17.5, 5) -> (-12.5, 5)
  line L140 (-12.5, 10) -> (-17.5, 10)
  line L141 (-12.5, 5) -> (-12.5, 10)
  line L142 (-10, 10) -> (-10, 5)
  line L143 (-10, 5) -> (-5, 5)
  line L144 (-5, 10) -> (-10, 10)
  line L145 (-5, 5) -> (-5, 10)
  line L146 (-2.5, 10) -> (-2.5, 5)
  line L147 (-2.5, 5) -> (2.5, 5)
  line L148 (2.5, 10) -> (-2.5, 10)
  line L149 (2.5, 5) -> (2.5, 10)
  line L150 (5, 10) -> (5, 5)
  line L151 (5, 5) -> (10, 5)
  line L152 (10, 10) -> (5, 10)
  line L153 (10, 5) -> (10, 10)
  line L154 (12.5, 10) -> (12.5, 5)
  line L155 (12.5, 5) -> (17.5, 5)
  line L156 (17.5, 10) -> (12.5, 10)
  line L157 (17.5, 5) -> (17.5, 10)
  line L158 (20, 10) -> (20, 5)
  line L159 (20, 5) -> (25, 5)
  line L160 (25, 10) -> (20, 10)
  line L161 (25, 5) -> (25, 10)
  line L162 (27.5, 10) -> (27.5, 5)
  line L163 (27.5, 5) -> (29.5804, 5)
  line L164 (28.2843, 10) -> (27.5, 10)
  line L165 (-25, 16.5831) -> (-25, 12.5)
  line L166 (-25, 12.5) -> (-20, 12.5)
  line L167 (-20, 17.5) -> (-24.367, 17.5)
  line L168 (-20, 12.5) -> (-20, 17.5)
  line L169 (-17.5, 17.5) -> (-17.5, 12.5)
  line L170 (-17.5, 12.5) -> (-12.5, 12.5)
  line L171 (-12.5, 17.5) -> (-17.5, 17.5)
  line L172 (-12.5, 12.5) -> (-12.5, 17.5)
  line L173 (-10, 17.5) -> (-10, 12.5)
  line L174 (-10, 12.5) -> (-5, 12.5)
  line L175 (-5, 17.5) -> (-10, 17.5)
  line L176 (-5, 12.5) -> (-5, 17.5)
  line L177 (-2.5, 17.5) -> (-2.5, 12.5)
  line L178 (-2.5, 12.5) -> (2.5, 12.5)
  line L179 (2.5, 17.5) -> (-2.5, 17.5)
  line L180 (2.5, 12.5) -> (2.5, 17.5)
  line L181 (5, 17.5) -> (5, 12.5)
  line L182 (5, 12.5) -> (10, 12.5)
  line L183 (10, 17.5) -> (5, 17.5)
  line L184 (10, 12.5) -> (10, 17.5)
  line L185 (12.5, 17.5) -> (12.5, 12.5)
  line L186 (12.5, 12.5) -> (17.5, 12.5)
  line L187 (17.5, 17.5) -> (12.5, 17.5)
  line L188 (17.5, 12.5) -> (17.5, 17.5)
  line L189 (20, 17.5) -> (20, 12.5)
  line L190 (20, 12.5) -> (25, 12.5)
  line L191 (24.367, 17.5) -> (20, 17.5)
  line L192 (25, 12.5) -> (25, 16.5831)
  line L193 (-22.3607, 20) -> (-20, 20)
  line L194 (-20, 20) -> (-20, 22.3607)
  line L195 (-17.5, 24.367) -> (-17.5, 20)
  line L196 (-17.5, 20) -> (-12.5, 20)
  line L197 (-12.5, 25) -> (-16.5831, 25)
  line L198 (-12.5, 20) -> (-12.5, 25)
  line L199 (-10, 25) -> (-10, 20)
  line L200 (-10, 20) -> (-5, 20)
  line L201 (-5, 25) -> (-10, 25)
  line L202 (-5, 20) -> (-5, 25)
  line L203 (-2.5, 25) -> (-2.5, 20)
  line L204 (-2.5, 20) -> (2.5, 20)
  line L205 (2.5, 25) -> (-2.5, 25)
  line L206 (2.5, 20) -> (2.5, 25)
  line L207 (5, 25) -> (5, 20)
  line L208 (5, 20) -> (10, 20)
  line L209 (10, 25) -> (5, 25)
  line L210 (10, 20) -> (10, 25)
  line L211 (12.5, 25) -> (12.5, 20)
  line L212 (12.5, 20) -> (17.5, 20)
  line L213 (16.5831, 25) -> (12.5, 25)
  line L214 (17.5, 20) -> (17.5, 24.367)
  line L215 (20, 22.3607) -> (20, 20)
  line L216 (20, 20) -> (22.3607, 20)
  line L217 (-10, 28.2843) -> (-10, 27.5)
  line L218 (-10, 27.5) -> (-5, 27.5)
  line L219 (-5, 27.5) -> (-5, 29.5804)
  line L220 (-2.5, 29.8957) -> (-2.5, 27.5)
  line L221 (-2.5, 27.5) -> (2.5, 27.5)
  line L222 (2.5, 27.5) -> (2.5, 29.8957)
  line L223 (5, 29.5804) -> (5, 27.5)
  line L224 (5, 27.5) -> (10, 27.5)
  line L225 (10, 27.5) -> (10, 28.2843)
  dimension "d27" = 210.25
  dimension "d28" = 60
  dimension "d29" = 5
  dimension "d30" = 5
  constraint coincident A0.centre A1.centre
  constraint concentric A0 A1
  constraint horizontal L0
  constraint perpendicular L0 L1
  constraint parallel L0 L2
  constraint parallel L1 L3
  constraint coincident L4 A0.centre
  constraint coincident L5 A0.centre
  constraint coincident A1 L217.start
  constraint coincident A1 L219.end
  constraint coincident A1 L220.start
  constraint coincident A1 L222.end
  constraint coincident A1 L223.start
  constraint coincident A1 L225.end
  constraint coincident A1 L194.end
  constraint coincident A1 L193.start
  constraint coincident A1 L167.end
  constraint coincident A1 L165.start
  constraint coincident A1 L197.end
  constraint coincident A1 L195.start
  constraint coincident A1 L132.end
  constraint coincident A1 L131.start
  constraint coincident A1 L102.end
  constraint coincident A1 L101.start
  constraint coincident A1 L68.end
  constraint coincident A1 L67.start
  constraint coincident A1 L39.end
  constraint coincident A1 L40.start
  constraint coincident A1 L15.end
  constraint coincident A1 L16.start
  constraint coincident A1 L17.end
  constraint coincident A1 L18.start
  constraint coincident A1 L6.end
  constraint coincident A1 L8.start
  constraint coincident A1 L9.end
  constraint coincident A1 L11.start
  constraint coincident A1 L12.end
  constraint coincident A1 L14.start
  constraint coincident A1 L34.end
  constraint coincident A1 L36.start
  constraint coincident A1 L37.end
  constraint coincident A1 L38.start
  constraint coincident A1 L66.start
  constraint coincident A1 L64.end
  constraint coincident A1 L100.start
  constraint coincident A1 L99.end
  constraint coincident A1 L130.start
  constraint coincident A1 L129.end
  constraint coincident A1 L163.end
  constraint coincident A1 L164.start
  constraint coincident A1 L191.start
  constraint coincident A1 L192.end
  constraint coincident A1 L216.end
  constraint coincident A1 L215.start
  constraint coincident A1 L213.start
  constraint coincident A1 L214.end
  measures "d27" diameter of A0
  measures "d28" diameter of A1
  measures "d29" distance of L1.end L2.end
  measures "d30" distance of L0.end L1.end
extrude "Extrude2" add sketch "Sketch4" along normal mid plane 8 separate body contours A1 L6 L7 L8 L9 L10 L11 L12 L13 L14 L15 L16 L17 L18 L19 L20 L33 L34 L35 L36 L37 L38 L39 L40 L41 L42 L63 L64 L65 L66 L67 L68 L69 L98 L99 L100 L101 L102 L103 L128 L129 L130 L131 L132 L133 L162 L163 L164 L165 L166 L167 L168 L189 L190 L191 L192 L193 L194 L195 L196 L197 L198 L211 L212 L213 L214 L215 L216 L217 L218 L219 L220 L221 L222 L223 L224 L225 makes body 2
revolve "Revolve2" add sketch "Sketch5" angle 360 about axis through (0, 0, 0) along (0, 0, 1) bodies 1 2
chamfer "Chamfer1" distance 3 angle 45 1 edges at (-97.8944, 37.9696, 200) on bodies 1
equation "d8 = ( 210 / 2 ) * 1 mm"
equation "d27 = ( ( ( 220 - 5 ) + ( 210.5 - 5 ) ) / 2 ) * 1 mm"

design "FA7 - 22-16 Gauge Heat Shrink Solder Seal"
Autodesk Fusion 360 part; units mm, degrees
sketch "Sketch1" plane through (0, 0, 0) normal (0, 0, 1) x (1, 0, 0)
  circle A0 centre (0, 0) radius 0.6455
  circle A1 centre (0, 0) radius 0.7
  dimension "d1" = 1.291
  dimension "d2" = 1.4
  constraint coincident A0.centre A1.centre
  measures "d1" diameter of A0
  measures "d2" diameter of A1
extrude "Extrude1" add sketch "Sketch1" along normal blind 12 makes body 1
sketch "Sketch2" plane through (0, 0, 0) normal (0, 0, 1) x (1, 0, 0)
  circle A0 centre (0, 0) radius 0.7
  circle A1 centre (0, 0) radius 0.75
  dimension "d5" = 1.4
  dimension "d6" = 1.5
  constraint coincident A0.centre A1.centre
  measures "d5" diameter of A0
  measures "d6" diameter of A1
extrude "Extrude2" add sketch "Sketch2" along normal blind 1 from surface at 2 separate body makes body 2
extrude "Extrude3" add sketch "Sketch2" against normal blind 1 from surface at 10 separate body makes body 3
extrude "Extrude4" add sketch "Sketch2" along normal mid plane 1 from surface at 6 separate body makes body 4

design "Lever (LB6)"
Autodesk Fusion 360 part; units mm, degrees
sketch "Sketch1" plane through (0, 0, 0) normal (0, 0, 1) x (1, 0, 0)
  circle A0 centre (0, 0) radius 1.5
  dimension "d1" = 3
  constraint coincident A0.centre origin
  measures "d1" diameter of A0
extrude "Extrude1" add sketch "Sketch1" along normal blind 28 makes body 1
sketch "Sketch2" plane through (0, 0, 28) normal (0, 0, 1) x (-1, 0, 0)
  circle A0 centre (0, 0) radius 1.5
  circle A1 centre (0, 0) radius 3
  dimension "d4" = 6
  constraint coincident A0.centre A1.centre
  measures "d4" diameter of A1
extrude "Extrude2" add sketch "Sketch2" along normal blind 2 contours A0 | A1 bodies 1
sketch "Sketch3" plane through (0, 0, 30) normal (0, 0, 1) x (-1, 0, 0)
  circle A0 centre (0, 0) radius 3
  line L0 (0, -3.5) -> (3.0311, -1.75)
  line L1 (3.0311, -1.75) -> (3.0311, 1.75)
  line L2 (3.0311, 1.75) -> (0, 3.5)
  line L3 (0, 3.5) -> (-3.0311, 1.75)
  line L4 (-3.0311, 1.75) -> (-3.0311, -1.75)
  line L5 (-3.0311, -1.75) -> (0, -3.5)
  dimension "d7" = 3.5
  constraint coincident A0.centre origin
  constraint vertical L4
  measures "d7" distance of L0.start A0.centre
extrude "Extrude3" add sketch "Sketch3" along normal blind 10 contours A0 | L0 L1 L2 L3 L4 L5 bodies 1